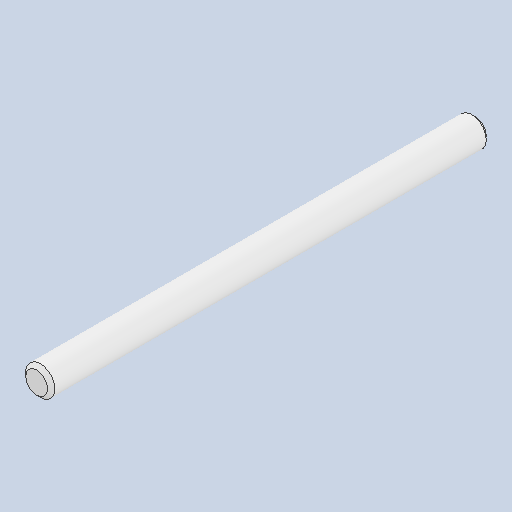
# Autodesk Inventor part: MotorBeltTensionerGuide
Saved by Autodesk Inventor 2023 (Build 270158000, 158)
## iProperties
Created: 2022-01-06
Part Number: MotorBeltTensionerGuide
Material: Generic
Document SubType Name: Modeling
Designer: Jochen
Density: 1 g/cm^3
Appearance: Default
Author: Jochen
Autodesk Inventor part; units mm, degrees
ref_plane "YZ Plane" through (0, 0, 0) normal (1, 0, 0) x (0, 1, 0)
ref_plane "XZ Plane" through (0, 0, 0) normal (0, 1, 0) x (-1, 0, 0)
ref_plane "XY Plane" through (0, 0, 0) normal (0, 0, 1) x (1, 0, 0)
sketch "Sketch1" plane through (0, 0, 0) normal (0, 0, 1) x (1, 0, 0)
  circle A0 centre (0, 0) radius 1
  dimension "d6" = 2
  constraints: 1 centre point
  measures "d6" diameter of A0
extrude "Extrusion2" add sketch "Sketch1" along normal blind 30
chamfer "Chamfer1" distance 0.25 angle 45 2 edges at (-1, 0, 0) (-1, 0, 30)
body "Solid1"
body "Solid2"
